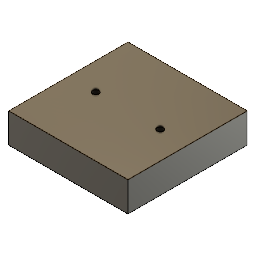
switch (Autodesk Fusion 360 design; units mm, degrees)
Autodesk Fusion 360 part; units mm, degrees
sketch "Sketch1" plane through (0, 0, 0) normal (0, 1, 0) x (1, 0, 0)
  line L0 (0, 0) -> (0, 100)
  line L1 (0, 100) -> (-100, 100)
  line L2 (-100, 100) -> (-100, 0)
  line L3 (-100, 0) -> (0, 0)
  dimension "d1" = 100
  dimension "d2" = 100
  dimension "d3" = 100
extrude "Extrude1" add sketch "Sketch1" along normal blind 25
sketch "Sketch2" plane through (0, 25, 0) normal (0, 1, 0) x (-1, 0, 0)
  line L0 (100, 0) -> (0, 0)
  line L1 (0, 0) -> (0, -100)
  line L2 (0, -100) -> (100, -100)
  line L3 (100, -100) -> (100, 0)
  circle A0 centre (23, -50) radius 2.5
  circle A1 centre (77, -50) radius 2.5
  dimension "d6" = 5
  dimension "d7" = 5
  dimension "d8" = 23
  dimension "d9" = 23
  dimension "d10" = 50
  dimension "d11" = 50
  dimension "d14" = 54
  measures "d6" diameter of A0
  measures "d7" diameter of A1
extrude "Extrude2" cut sketch "Sketch2" against normal blind 90 contours A0 | A1
